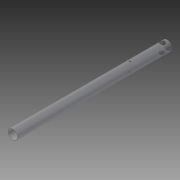
# Autodesk Inventor part: Polycarbonate Clamp Tube 1 in OD (8585K14)
Saved by Autodesk Inventor 2014 SP1 (Build 180222100, 222)
## iProperties
Created: 2014-01-13
Part Number: Polycarbonate Clamp Tube 1 in OD (8585K14)
Material: Polycarbonate, Clear
Document SubType Name: Modeling
Designer: Michael
Density: 1.2 g/cm^3
Appearance: Polycarbonate - Clear
Mass: 55.9655 g
Surface Area: 590.918 cm^2
Volume: 46.6379 cm^3
Author: Michael
Autodesk Inventor part; units mm, degrees
ref_plane "YZ Plane" through (0, 0, 0) normal (1, 0, 0) x (0, 1, 0)
ref_plane "XY Plane" through (0, 0, 0) normal (0, 0, 1) x (1, 0, 0)
sketch "Sketch1" plane through (0, 0, 0) normal (0, 0, 1) x (1, 0, 0)
  circle A0 centre (0, 0) radius 12.7
  circle A1 centre (0, 0) radius 11.1125
  dimension "d0" = 25.4
  dimension "d1" = 22.225
  constraints: 2 centre point, 2 coincident
  measures "d0" diameter of A0
  measures "d1" diameter of A1
extrude "Extrusion1" add sketch "Sketch1" along normal blind 393.7
ref_plane "Work Plane1" through (0, 12.7, 0) normal (0, 1, 0) x (-1, 0, 0)
sketch "Sketch2" plane through (0, 12.7, 0) normal (0, 1, 0) x (-1, 0, 0)
  line L0 (-12.7, 0) -> (-12.7, 393.7) projected
  line L1 (-12.7, 0) -> (12.7, 0) projected
  line L2 (12.7, 0) -> (12.7, 393.7) projected
  circle A0 centre (0, 12.7) radius 6.35
  line L3 (0, 0) -> (0, 58.059) construction
  circle A1 centre (0, 95.25) radius 2.413
  dimension "d4" = 12.7
  dimension "d6" = 12.7
  dimension "d10" = 4.826
  dimension "d11" = 95.25
  constraints: 2 centre point, 2 end point, 2 point on line, 1 parallel
  measures "d4" diameter of A0
  measures "d6" distance from line of L1 A0.centre
  measures "d10" diameter of A1
  measures "d11" distance from line of L1 A1.centre
extrude "Extrusion2" cut sketch "Sketch2" against normal blind 25.4
body "Solid1"
